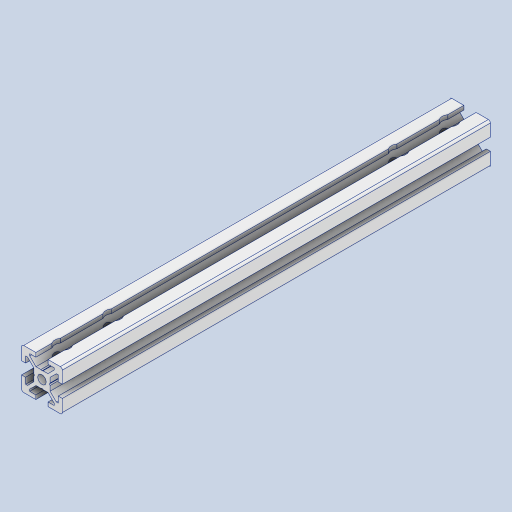
# Autodesk Inventor part: HFS5-2020-210-AV10-BV35-CV175-DV200
Saved by Autodesk Inventor 2023 (Build 270158000, 158)
## iProperties
Category: PARTsolutions
Company: MISUMI
Created: 2024-11-20
Part Number: HFS5-2020-210-AV10-BV35-CV175-DV200
Material: アルミニウム 6061
Catalog Web Link: www.cadenas.de
Description: NFS5-2020, NFSB5-2020, HFS5-2020, HFSB5-2020, CAF5-2020, HFSY5-2020, NFSF5-2020, HFSF5-2020, HFSFB5-2020, NFST5-2020, HFST5-2020, HFSTB5-2020, HFSH5-2020, HFSC5-2020-HFS5 Series Aluminum Extrusions 20 Square -1 Slot-
Vendor: MISUMI
Document SubType Name: Modeling
Designer: psAdmin
Manufacturer: MISUMI
Mass: 100.485 g
Surface Area: 367.434 cm^2
Volume: 37.2166 cm^3
Density: 2.7 g/cm^3
Appearance: アルミニウム - フラット
PSOL_IDENT_0: {$CADENAS_DATA/23d-libs/misumi/metric/38_al_extrusions_blackets/5/hfs5_2020.prj},721 {VTYP=3D},{NB=H
PSOL_IDENT_1: FS5-2020-210-AV10-BV35-CV175-DV200},{LINA=HFS5-2020-210-AV10-BV35-CV175-DV200},{NN=NFS5-2020, NFSB5-
PSOL_IDENT_2: 2020, HFS5-2020, HFSB5-2020, CAF5-2020, HFSY5-2020, NFSF5-2020, HFSF5-2020, HFSFB5-2020, NFST5-2020,
PSOL_IDENT_3: HFST5-2020, HFSTB5-2020, HFSH5-2020, HFSC5-2020},{DATE=08.05.2023 08:39:06},{GEOMDATE=27.07.2021 03
PSOL_IDENT_4: :20:00},{VERSION=},{LINEID=150},{WBVAR=L,ALT1,ALT2,ALT4,ALT5,CP5,DL5,DR5,ALT6,ALT9,ALT10,ALT11,HP6,N
PSOL_IDENT_5: HL6,DL6,NHR6,DR6,ALT7,ALT8,NH9,AH,BH,CH,DH,EH,NH10,AV,BV,CV,DV,EV,NH11,AP,BP,CP,DP,EP,ALT12,ALT13,Z,
PSOL_IDENT_6: NH12,XA,XB,XC,XD,XE,NH13,YA,YB,YC,YD,YE,ALT16,HP16,DL16,DR16,ALT17,HQ17,JLP,ALT20},{WBNUMERIC=L,NH9,
PSOL_IDENT_7: AH,BH,CH,DH,EH,NH10,AV,BV,CV,DV,EV,NH11,AP,BP,CP,DP,EP,NH12,XA,XB,XC,XD,XE,NH13,YA,YB,YC,YD,YE,HQ17,
PSOL_IDENT_8: JLP}  {NB=HFS5-2020-210-AV10-BV35-CV175-DV200},{LINA=HFS5-2020-210-AV10-BV35-CV175-DV200},{KT=DUMMY}
PSOL_IDENT_9: ,{PN=HFS5-2020-210-AV10-BV35-CV175-DV200},{TPS=HFS5-2020},{MAT=A6N01SS-T5 Aluminum Alloy or 6005A-T5
PSOL_IDENT_10: Aluminum Alloy},{ST=Clear Anodize},{FRMW=20},{FRMH=20},{FRD=4.2},{L=210},{MASS=0.5},{SA=183},{LX=0.
PSOL_IDENT_11: 742x10^4},{LY=0.742x10^4},{ALT1=},{M1=0},{DPL1=0},{DPR1=0},{ALT1PN=},{ALT2=},{ALT2ALG= '','w/o End T
PSOL_IDENT_12: apping (Heli-Coil Insert)','LHP','with LHP (Tapping on the Left (Heli-Coil Insert))','RHP','with RHP
PSOL_IDENT_13: (Tapping on the Right (Heli-Coil Insert))','HPW','with HPW (Tapping on Both Ends (Heli-Coil Insert)
PSOL_IDENT_14: )' },{M2=0},{DP2=0},{ALT2PN=},{ALT4=},{ALT4ALG= '', 'w/o SC (High Precision Cut)', 'SC', 'with SC (H
PSOL_IDENT_15: igh Precision Cut)' },{ALT4PN=},{ALT5=},{ALT5ALG= '','w/o 45 Degree Cut','1','with 45 Degree Cut' },
PSOL_IDENT_16: {CP5=},{CP5ALG= '','N/A' },{DL5=},{DL5ALG= '','N/A' },{DR5=},{DR5ALG= '','N/A' },{FRMLALT5=0},{FRMRA
PSOL_IDENT_17: LT5=0},{ALT5PN=},{ALT6=},{ALT6ALG= '','w/o Fastening Location Wrench Access Hole Alterations','1','w
PSOL_IDENT_18: ith Fastening Location Wrench Access Hole Alterations' },{ALT9=},{ALT9ALG= '','w/o Location Specifie
PSOL_IDENT_19: d Wrench Access Hole Alteratons (Horizontal)','1','with Location Specified Wrench Access Hole Altera
PSOL_IDENT_20: tons (Horizontal)' },{ALT10=1},{ALT10ALG= '','w/o Location Specified Wrench Access Hole Alteratons (
PSOL_IDENT_21: Vertical)','1','with Location Specified Wrench Access Hole Alteratons (Vertical)' },{ALT11=},{ALT11A
PSOL_IDENT_22: LG= '','w/o Location Specified Wrench Access Hole Alteratons (Crisscross)','1','with Location Specif
PSOL_IDENT_23: ied Wrench Access Hole Alteratons (Crisscross)' },{HP6=},{HP6ALG= '','N/A' },{NHL6=},{NHL6ALG= '','N
PSOL_IDENT_24: /A' },{DL6=},{DL6ALG= '','N/A' },{NHR6=},{NHR6ALG= '','N/A' },{DR6=},{DR6ALG= '','N/A' },{HL6=0.000}
PSOL_IDENT_25: ,{HL6D=0},{HR6=0.000},{HR6D=0},{J6=0},{J6D=0},{K6=0},{K6D=0},{DD6=7.35},{DD6ALG=7.35},{ALT7=},{ALT7A
PSOL_IDENT_26: LG= '','N/A' },{ALT8=},{ALT8ALG= '','N/A' },{ALT678PN=},{NH9=0},{NH9MAX=5},{NH9ALG=[0]},{AH=0.0},{AH
PSOL_IDENT_27: MIN=7},{AHMAX=212.5},{AHALG=[0]},{BH=0.0},{BHMIN=9.5},{BHMAX=222},{BHALG=[0]},{CH=0.0},{CHMIN=9.5},{
PSOL_IDENT_28: CHMAX=231.5},{CHALG=[0]},{DH=0.0},{DHMIN=9.5},{DHMAX=241},{DHALG=[0]},{EH=0.0},{EHMIN=9.5},{EHMAX=20
PSOL_IDENT_29: 3},{EHALG=[0]},{NH10=4},{NH10MAX=5},{NH10ALG=[1:5/1]},{AV=10.0},{AVMIN=7},{AVMAX=174.5},{AVALG=[7:17
PSOL_IDENT_30: 4.5/0.5]},{BV=35.0},{BVMIN=19.5},{BVMAX=184},{BVALG=[19.5:184/0.5]},{CV=175.0},{CVMIN=44.5},{CVMAX=1
PSOL_IDENT_31: 93.5},{CVALG=[44.5:193.5/0.5]},{DV=200.0},{DVMIN=184.5},{DVMAX=203},{DVALG=[184.5:203/0.5]},{EV=0.0}
PSOL_IDENT_32: ,{EVMIN=209.5},{EVMAX=203},{EVALG=[0]},{NH11=0},{NH11MAX=5},{NH11ALG=[0]},{AP=0.0},{APMIN=7},{APMAX=
PSOL_IDENT_33: 212.5},{APALG=[0]},{BP=0.0},{BPMIN=9.5},{BPMAX=222},{BPALG=[0]},{CP=0.0},{CPMIN=9.5},{CPMAX=231.5},{
PSOL_IDENT_34: CPALG=[0]},{DP=0.0},{DPMIN=9.5},{DPMAX=241},{DPALG=[0]},{EP=0.0},{EPMIN=9.5},{EPMAX=203},{EPALG=[0]}
PSOL_IDENT_35: ,{ALT9PN=},{ALT10PN=-AV10-BV35-CV175-DV200},{ALT11PN=},{ALT91011PN=-AV10-BV35-CV175-DV200},{ALT12=},
PSOL_IDENT_36: {ALT12ALG= '','w/o Counterbore Hole in Specified Position (Vertical)','1','with Counterbore Hole in
PSOL_IDENT_37: Specified Position (Vertical)' },{ALT13=},{ALT13ALG= '','w/o Counterbore Hole in Specified Position
PSOL_IDENT_38: (Horizontal)','1','with Counterbore Hole in Specified Position (Horizontal)' },{Z=},{ZALG= '','N/A'
PSOL_IDENT_39: },{DD12=0.0},{DD112=0.0},{NH12=0},{NH12MAX=5},{NH12ALG=[0]},{XA=0.0},{XAMIN=7},{XAMAX=205},{XAALG=[0
PSOL_IDENT_40: ]},{XB=0.0},{XBMIN=2},{XBMAX=207},{XBALG=[0]},{XC=0.0},{XCMIN=2},{XCMAX=209},{XCALG=[0]},{XD=0.0},{X
PSOL_IDENT_41: DMIN=2},{XDMAX=211},{XDALG=[0]},{XE=0.0},{XEMIN=2},{XEMAX=203},{XEALG=[0]},{NH13=0},{NH13MAX=5},{NH1
PSOL_IDENT_42: 3ALG=[0]},{YA=0.0},{YAMIN=7},{YAMAX=205},{YAALG=[0]},{YB=0.0},{YBMIN=2},{YBMAX=207},{YBALG=[0]},{YC=
PSOL_IDENT_43: 0.0},{YCMIN=2},{YCMAX=209},{YCALG=[0]},{YD=0.0},{YDMIN=2},{YDMAX=211},{YDALG=[0]},{YE=0.0},{YEMIN=2}
PSOL_IDENT_44: ,{YEMAX=203},{YEALG=[0]},{ALT12PN=},{ALT13PN=},{ALT1213PN=},{ALT16=},{ALT16ALG= '','w/o M Type Hole
PSOL_IDENT_45: Alteration','1','with M Type Hole Alteration' },{HP16=},{HP16ALG= '','N/A' },{DL16=},{DL16ALG= '','N
PSOL_IDENT_46: /A' },{DR16=},{DR16ALG= '','N/A' },{H116=0},{D16=0.0},{ALT16PN=},{ALT17=},{ALT17ALG= '','w/o L Type
PSOL_IDENT_47: Hole Alteration (Top)','1','with L Type Hole Alteration (Top)' },{HQ17=0},{HQ17ALG=0},{JLP=0},{JLPMI
PSOL_IDENT_48: N=4.9},{JLPMAX=0},{JLPALG=[0]},{L17=0},{D17=0.0},{ALT17PN=},{ALT20=},{ALT20PN=},{ERRORALT01=OK},{ERR
PSOL_IDENT_49: ORALT02=OK},{ERRORALT05=OK},{ERRORALT06091=OK},{ERRORALT06092=OK},{ERRORALT06093=OK},{ERRORALT06094=
PSOL_IDENT_50: OK},{ERRORALT06101=OK},{ERRORALT06102=OK},{ERRORALT06103=OK},{ERRORALT06104=OK},{ERRORALT06111=OK},{
PSOL_IDENT_51: ERRORALT06112=OK},{ERRORALT06113=OK},{ERRORALT06114=OK},{ERRORALT06121=OK},{ERRORALT06122=OK},{ERROR
PSOL_IDENT_52: ALT06123=OK},{ERRORALT06124=OK},{ERRORALT06131=OK},{ERRORALT06132=OK},{ERRORALT06133=OK},{ERRORALT06
PSOL_IDENT_53: 134=OK},{ERRORALT0616=OK},{ERRORALT06171=OK},{ERRORALT06172=OK},{ERRORALT06173=OK},{ERRORALT0911=OK}
PSOL_IDENT_54: ,{ERRORALT0913=OK},{ERRORALT0916=OK},{ERRORALT0917=OK},{ERRORALT1011=OK},{ERRORALT1012=OK},{ERRORALT
PSOL_IDENT_55: 1016=OK},{ERRORALT1017=OK},{ERRORALT1112=OK},{ERRORALT1113=OK},{ERRORALT1116=OK},{ERRORALT1117=OK},{
PSOL_IDENT_56: ERRORALT1216=OK},{ERRORALT1217=OK},{ERRORALT1316=OK},{ERRORALT1317=OK},{ERRORALT1617=OK},{ERRORPN=},
PSOL_IDENT_57: {TFW=0}
NB: HFS5-2020-210-AV10-BV35-CV175-DV200
NN: NFS5-2020, NFSB5-2020, HFS5-2020, HFSB5-2020, CAF5-2020, HFSY5-2020, NFSF5-2020, HFSF5-2020, HFSFB5-2020, NFST5-2020, HFST5-2020, HFSTB5-2020, HFSH5-2020, HFSC5-2020
NT: HFS5 Series Aluminum Extrusions 20 Square -1 Slot-
NBSYN: $PN.
LINA: HFS5-2020-210-AV10-BV35-CV175-DV200
CATALOG: Misumi
PN: HFS5-2020-210-AV10-BV35-CV175-DV200
TPS: HFS5-2020
MAT: A6N01SS-T5 Aluminum Alloy or 6005A-T5 Aluminum Alloy
ST: Clear Anodize
L: 210
MASS: 0.5
SA: 183
LX: 0.742x10^4
LY: 0.742x10^4
ALT1: w/o End Tapping
M1: 0
DPL1: 0
DPR1: 0
ALT2: w/o End Tapping (Heli-Coil Insert)
M2: 0
DP2: 0
ALT4: w/o SC (High Precision Cut)
ALT5: w/o 45 Degree Cut
CP5: N/A
DL5: N/A
DR5: N/A
ALT6: w/o Fastening Location Wrench Access Hole Alterations
ALT9: w/o Location Specified Wrench Access Hole Alteratons (Horizontal)
ALT10: with Location Specified Wrench Access Hole Alteratons (Vertical)
ALT11: w/o Location Specified Wrench Access Hole Alteratons (Crisscross)
HP6: N/A
NHL6: N/A
DL6: N/A
NHR6: N/A
DR6: N/A
HL6D: 0
HR6D: 0
J6D: 0
K6D: 0
DD6: 7.35
ALT7: N/A
ALT8: N/A
NH9: 0
AH: 0
BH: 0
CH: 0
DH: 0
EH: 0
NH10: 4
AV: 10
BV: 35
CV: 175
DV: 200
EV: 0
NH11: 0
AP: 0
BP: 0
CP: 0
DP: 0
EP: 0
ALT12: w/o Counterbore Hole in Specified Position (Vertical)
ALT13: w/o Counterbore Hole in Specified Position (Horizontal)
Z: N/A
DD12: 0
DD112: 0
NH12: 0
XA: 0
XB: 0
XC: 0
XD: 0
XE: 0
NH13: 0
YA: 0
YB: 0
YC: 0
YD: 0
YE: 0
ALT16: w/o M Type Hole Alteration
HP16: N/A
DL16: N/A
DR16: N/A
H116: 0
D16: 0
ALT17: w/o L Type Hole Alteration (Top)
HQ17: 0
JLP: 0
D17: 0
ALT20: w/o CW (End Face C Chamfering)
SUPPLIER: MISUMI
ARTICLENO: HFS5-2020-210-AV10-BV35-CV175-DV200
BOMINFO: HFS5-2020-210-AV10-BV35-CV175-DV200
CREATOR: CADENAS GmbH
Title: HFS5-2020-210-AV10-BV35-CV175-DV200
Author: Cadenas PARTsolutions
Comments: HFS5 Series Aluminum Extrusions 20 Square -1 Slot-
Autodesk Inventor part; units mm, degrees
sketch "Sketch_1" plane through (0, 0, 0) normal (0, 0, 1) x (1, 0, 0)
  line L0 (-10, -3) -> (-10, -9)
  arc A0 (-10, -9) -> (-9, -10) centre (-9, -9) ccw
  line L1 (-9, -10) -> (-3, -10)
  line L2 (-3, -10) -> (-3, -8)
  line L3 (-3, -8) -> (-6, -8)
  line L4 (-6, -8) -> (-6, -7.0607)
  line L5 (-6, -7.0607) -> (-2.9393, -4)
  line L6 (-2.9393, -4) -> (-0.5196, -4)
  line L7 (-0.5196, -4) -> (0, -3.7)
  line L8 (0, -3.7) -> (0.5196, -4)
  line L9 (0.5196, -4) -> (2.9393, -4)
  line L10 (2.9393, -4) -> (6, -7.0607)
  line L11 (6, -7.0607) -> (6, -8)
  line L12 (6, -8) -> (3, -8)
  line L13 (3, -8) -> (3, -10)
  line L14 (3, -10) -> (9, -10)
  arc A1 (9, -10) -> (10, -9) centre (9, -9) ccw
  line L15 (10, -9) -> (10, -3)
  line L16 (10, -3) -> (8, -3)
  line L17 (8, -3) -> (8, -6)
  line L18 (8, -6) -> (7.0607, -6)
  line L19 (7.0607, -6) -> (4, -2.9393)
  line L20 (4, -2.9393) -> (4, -0.5196)
  line L21 (4, -0.5196) -> (3.7, 0)
  line L22 (3.7, 0) -> (4, 0.5196)
  line L23 (4, 0.5196) -> (4, 2.9393)
  line L24 (4, 2.9393) -> (7.0607, 6)
  line L25 (7.0607, 6) -> (8, 6)
  line L26 (8, 6) -> (8, 3)
  line L27 (8, 3) -> (10, 3)
  line L28 (10, 3) -> (10, 9)
  arc A2 (10, 9) -> (9, 10) centre (9, 9) ccw
  line L29 (9, 10) -> (3, 10)
  line L30 (3, 10) -> (3, 8)
  line L31 (3, 8) -> (6, 8)
  line L32 (6, 8) -> (6, 7.0607)
  line L33 (6, 7.0607) -> (2.9393, 4)
  line L34 (2.9393, 4) -> (0.5196, 4)
  line L35 (0.5196, 4) -> (0, 3.7)
  line L36 (0, 3.7) -> (-0.5196, 4)
  line L37 (-0.5196, 4) -> (-2.9393, 4)
  line L38 (-2.9393, 4) -> (-6, 7.0607)
  line L39 (-6, 7.0607) -> (-6, 8)
  line L40 (-6, 8) -> (-3, 8)
  line L41 (-3, 8) -> (-3, 10)
  line L42 (-3, 10) -> (-9, 10)
  arc A3 (-9, 10) -> (-10, 9) centre (-9, 9) ccw
  line L43 (-10, 9) -> (-10, 3)
  line L44 (-10, 3) -> (-8, 3)
  line L45 (-8, 3) -> (-8, 6)
  line L46 (-8, 6) -> (-7.0607, 6)
  line L47 (-7.0607, 6) -> (-4, 2.9393)
  line L48 (-4, 2.9393) -> (-4, 0.5196)
  line L49 (-4, 0.5196) -> (-3.7, 0)
  line L50 (-3.7, 0) -> (-4, -0.5196)
  line L51 (-4, -0.5196) -> (-4, -2.9393)
  line L52 (-4, -2.9393) -> (-7.0607, -6)
  line L53 (-7.0607, -6) -> (-8, -6)
  line L54 (-8, -6) -> (-8, -3)
  line L55 (-8, -3) -> (-10, -3)
  constraints: 112 end point, 8 point on circle, 4 centre point
extrude "Extrusion1" add sketch "Sketch_1" against normal blind 210
sketch "Sketch2" plane through (0, 0, -210) normal (0, 0, -1) x (-1, 0, 0)
  point P0 (0, 0)
hole "Hole1" at (0, 0, -210) direction (0, 0, 1) diameter 4.2 depth 210
sketch "Sketch_29" plane through (0, 0, 0) normal (1, 0, 0) x (0, 0, -1)
  line L0 (10, -10) -> (10, 10)
  line L1 (10, 10) -> (13.675, 10)
  line L2 (13.675, 10) -> (13.675, -10)
  line L3 (13.675, -10) -> (10, -10)
  line L4 (10, -10) -> (10, 10)
  constraints: 10 end point
revolve "Revolution1" cut sketch "Sketch_29" angle 360 about axis through (0, -10, -10) along (0, -1, 0)
sketch "Sketch_32" plane through (0, 0, 0) normal (1, 0, 0) x (0, 0, -1)
  line L0 (35, -10) -> (35, 10)
  line L1 (35, 10) -> (38.675, 10)
  line L2 (38.675, 10) -> (38.675, -10)
  line L3 (38.675, -10) -> (35, -10)
  line L4 (35, -10) -> (35, 10)
  constraints: 10 end point
revolve "Revolution2" cut sketch "Sketch_32" angle 360 about axis through (0, -10, -35) along (0, -1, 0)
sketch "Sketch_33" plane through (0, 0, 0) normal (1, 0, 0) x (0, 0, -1)
  line L0 (175, -10) -> (175, 10)
  line L1 (175, 10) -> (178.675, 10)
  line L2 (178.675, 10) -> (178.675, -10)
  line L3 (178.675, -10) -> (175, -10)
  line L4 (175, -10) -> (175, 10)
  constraints: 10 end point
revolve "Revolution3" cut sketch "Sketch_33" angle 360 about axis through (0, -10, -175) along (0, -1, 0)
sketch "Sketch_34" plane through (0, 0, 0) normal (1, 0, 0) x (0, 0, -1)
  line L0 (200, -10) -> (200, 10)
  line L1 (200, 10) -> (203.675, 10)
  line L2 (203.675, 10) -> (203.675, -10)
  line L3 (203.675, -10) -> (200, -10)
  line L4 (200, -10) -> (200, 10)
  constraints: 10 end point
revolve "Revolution4" cut sketch "Sketch_34" angle 360 about axis through (0, -10, -200) along (0, -1, 0)
ref_plane "C1_XY" through (0, 0, 0) normal (0, 0, 1) x (1, 0, 0)
ref_plane "C1_YZ" through (0, 0, 0) normal (1, 0, 0) x (0, 1, 0)
ref_plane "C1_ZX" through (0, 0, 0) normal (0, 1, 0) x (0, 0, 1)
body "Solid1"
